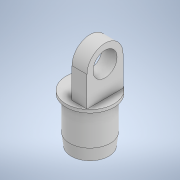
# Autodesk Inventor part: center_holder_top
Saved by Autodesk Inventor 2020 (Build 240168000, 168)
## iProperties
Created: 2019-04-30
Part Number: center_holder_top
Material: Generic
Document SubType Name: Modeling
Designer: erwin
Density: 1 g/cm^3
Appearance: Default
Author: erwin
Autodesk Inventor part; units mm, degrees
ref_plane "YZ Plane" through (0, 0, 0) normal (1, 0, 0) x (0, 1, 0)
ref_plane "XZ Plane" through (0, 0, 0) normal (0, 1, 0) x (-1, 0, 0)
ref_plane "XY Plane" through (0, 0, 0) normal (0, 0, 1) x (1, 0, 0)
sketch "Sketch1" plane through (0, 0, 0) normal (0, 1, 0) x (-1, 0, 0)
  circle A0 centre (0, 0) radius 6.75
  dimension "d0" = 13.5
  constraints: 1 centre point, 1 coincident
  measures "d0" diameter of A0
extrude "Extrusion1" add sketch "Sketch1" along normal blind 15
chamfer "Chamfer1" distance 4 distance2 0.5 1 edges at (6.75, 0, 0) measured on face at (-6.7281, 10, -0.5431)
sketch "Sketch2" plane through (0, 15, 0) normal (0, 1, 0) x (1, 0, 0)
  circle A0 centre (0, 0) radius 8
  dimension "d6" = 16
  constraints: 1 centre point, 1 coincident
  measures "d6" diameter of A0
extrude "Extrusion2" add sketch "Sketch2" along normal blind 1
sketch "Sketch3" plane through (0, 0, 0) normal (1, 0, 0) x (0, 1, 0)
  circle A0 centre (26, 0) radius 4
  arc A1 (26, -6) -> (26, 6) centre (26, 0) ccw
  line L0 (16, -8) -> (16, 8) projected
  line L1 (26, 6) -> (16, 6)
  line L2 (16, 6) -> (16, -6)
  line L3 (16, -6) -> (26, -6)
  point P0 (0, 0)
  dimension "d9" = 8
  dimension "d10" = 2
  dimension "d11" = 10
  constraints: 6 end point, 2 centre point, 2 point on circle, 1 horizontal, 1 parallel, 1 perpendicular, 1 point on line
  measures "d9" diameter of A0
  measures "d10" radial gap between concentric circles of A0 A1
  measures "d11" distance from line of L0 A0.centre
extrude "Extrusion3" add sketch "Sketch3" along normal blind 5
body "Solid1"
